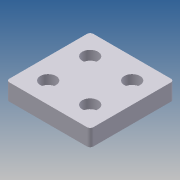
# Autodesk Inventor part: 21-8000Z1
Saved by Autodesk Inventor 2013 SP1 (Build 170176100, 176)
## iProperties
Created: 2011-01-07
Part Number: 21-8000Z1
Material: Aluminum-6061
Document SubType Name: Modeling
Designer: dc85560
Stock Number: Standard
Mass: 254.183 g
Surface Area: 197.638 cm^2
Volume: 93.7944 cm^3
Density: 2.71 g/cm^3
Title: Blank Plate 80x80
Author: dc85560
Autodesk Inventor part; units mm, degrees
ref_plane "YZ Plane" through (0, 0, 0) normal (1, 0, 0) x (0, 1, 0)
ref_plane "XZ Plane" through (0, 0, 0) normal (0, 1, 0) x (-1, 0, 0)
ref_plane "XY Plane" through (0, 0, 0) normal (0, 0, 1) x (1, 0, 0)
sketch "Sketch1" plane through (0, 0, 0) normal (0, 0, 1) x (1, 0, 0)
  line L0 (-40, 40) -> (40, 40)
  line L1 (40, 40) -> (40, -40)
  line L2 (40, -40) -> (-40, -40)
  line L3 (-40, -40) -> (-40, 40)
  point P0 (0, 0)
  dimension "d0" = 80
  dimension "d1" = 80
  dimension "d2" = 40
  dimension "d3" = 40
  constraints: 8 end point, 2 parallel, 1 horizontal, 1 perpendicular
  measures "d0" distance of L0.start L0.end
  measures "d1" distance of L2.end L0.start
  measures "d2" distance from line of point (0, 0) L3
  measures "d3" distance from line of point (0, 0) L0
extrude "Extrusion1" add sketch "Sketch1" against normal blind 15.9
sketch "Sketch2" plane through (0, 0, 0) normal (0, 0, 1) x (1, 0, 0)
  line L0 (0, 56) -> (0, -56) projected
  line L1 (-56, 0) -> (56, 0) projected
  point P0 (-20, 20)
  dimension "d6" = 20
  dimension "d7" = 20
  measures "d6" distance from line of L0 point (-20, 20)
  measures "d7" distance from line of L1 point (-20, 20)
hole "Hole1" at (-20, 20, 0) direction (0, 0, -1) diameter 8.4 end through all counterbore diameter 15 counterbore depth 8.9 clearance for "Socket Head Cap Screw" size "M8" standard "Ansi Metric M Profile"
mirror "Mirror1" about plane through (0, 0, 0) normal (1, 0, 0) of "Hole1"
mirror "Mirror2" about plane through (0, 0, 0) normal (0, 1, 0) of "Hole1", "Mirror1"
fillet "Fillet1" radius 3 4 edges at (-40, -40, -7.95) (-40, 40, -7.95) (40, 40, -7.95) (40, -40, -7.95)
equation "\"d2\" = 0.5 * d0"
equation "\"d3\" = d2"
equation "\"d7\" = d6"
body "Solid1"
